Autodesk Inventor part; units mm, degrees
(part 5 of 16)
  spline S25 degree 3 poles (-39.1458, 73.8476) (-39.0245, 73.9067) (-38.9024, 73.9639) (-38.7794, 74.0192) (-38.7128, 74.0491) (-38.6461, 74.0784) (-38.5791, 74.1071) (-38.5156, 74.1342) (-38.4519, 74.1608) (-38.388, 74.1869) (-38.3277, 74.2114) (-38.2671, 74.2355) (-38.2064, 74.259) (-38.1493, 74.2811) (-38.0919, 74.3027) (-38.0344, 74.3237) (-37.9806, 74.3435) (-37.9265, 74.3627) (-37.8723, 74.3815) (-37.8218, 74.399) (-37.7711, 74.4161) (-37.7203, 74.4327) (-37.6731, 74.4481) (-37.6259, 74.4631) (-37.5784, 74.4776) (-37.5348, 74.491) (-37.4909, 74.5041) (-37.447, 74.5167) (-37.4068, 74.5283) (-37.3665, 74.5395) (-37.3262, 74.5503) (-37.2895, 74.5602) (-37.2528, 74.5697) (-37.216, 74.5789) (-37.183, 74.5871) (-37.1499, 74.5951) (-37.1167, 74.6027) (-37.0728, 74.6128) (-37.0288, 74.6223) (-36.9848, 74.6314) (-36.9749, 74.6334) (-36.9651, 74.6354) (-36.9552, 74.6375) (-36.9456, 74.6396) (-36.936, 74.6418) (-36.9264, 74.6441) (-36.917, 74.6463) (-36.9077, 74.6485) (-36.8984, 74.6509) (-36.8892, 74.6532) (-36.8801, 74.6556) (-36.871, 74.6581) (-36.8621, 74.6606) (-36.8531, 74.6631) (-36.8443, 74.6657) (-36.8355, 74.6683) (-36.8268, 74.671) (-36.8181, 74.6738) (-36.8095, 74.6765) (-36.801, 74.6794) (-36.7925, 74.6823) (-36.7841, 74.6852) (-36.7757, 74.6882) (-36.7673, 74.6914) (-36.759, 74.6945) (-36.7507, 74.6977) (-36.7425, 74.7011) (-36.7342, 74.7044) (-36.726, 74.7079) (-36.7179, 74.7115) (-36.7096, 74.7151) (-36.7015, 74.7189) (-36.6934, 74.7228) (-36.6851, 74.7268) (-36.677, 74.7309) (-36.6689, 74.7351) (-36.6606, 74.7395) (-36.6523, 74.7441) (-36.6442, 74.7489) (-36.6357, 74.7538) (-36.6274, 74.7589) (-36.6191, 74.7642) (-36.6105, 74.7698) (-36.6019, 74.7757) (-36.5936, 74.7817) (-36.5846, 74.7882) (-36.5758, 74.795) (-36.5673, 74.802) (-36.558, 74.8097) (-36.5489, 74.8176) (-36.5402, 74.8259) (-36.5305, 74.835) (-36.5213, 74.8445) (-36.5124, 74.8544) (-36.5025, 74.8654) (-36.4931, 74.8769) (-36.4843, 74.8888) (-36.4745, 74.9022) (-36.4653, 74.9162) (-36.457, 74.9306) (-36.4476, 74.9468) (-36.4392, 74.9636) (-36.432, 74.9809) (-36.424, 75.0001) (-36.4175, 75.0199) (-36.4123, 75.0401) (-36.4067, 75.0619) (-36.4028, 75.0843) (-36.401, 75.1067) (-36.3992, 75.1282) (-36.3993, 75.1498) (-36.3998, 75.1713) (-36.4022, 75.2779) (-36.4136, 75.3839) (-36.4198, 75.4902) (-36.426, 75.5965) (-36.427, 75.7031) (-36.437, 75.8092) (-36.439, 75.8307) (-36.4414, 75.8521) (-36.4457, 75.8732) (-36.4501, 75.8953) (-36.4566, 75.9171) (-36.4647, 75.9381) (-36.4721, 75.9576) (-36.481, 75.9765) (-36.4911, 75.9946) (-36.5003, 76.0109) (-36.5105, 76.0267) (-36.5217, 76.0417) (-36.5317, 76.055) (-36.5424, 76.0678) (-36.5538, 76.08) (-36.5639, 76.0908) (-36.5745, 76.1011) (-36.5857, 76.1109) (-36.5956, 76.1197) (-36.6059, 76.1281) (-36.6166, 76.136) (-36.6262, 76.1432) (-36.6361, 76.1501) (-36.6462, 76.1566) (-36.6555, 76.1625) (-36.665, 76.1682) (-36.6747, 76.1736) (-36.6837, 76.1787) (-36.6929, 76.1835) (-36.7021, 76.1881) (-36.7109, 76.1924) (-36.7198, 76.1965) (-36.7288, 76.2004) (-36.7374, 76.2042) (-36.7461, 76.2078) (-36.7549, 76.2112) (-36.7635, 76.2145) (-36.7721, 76.2176) (-36.7807, 76.2206) (-36.7892, 76.2236) (-36.7977, 76.2263) (-36.8063, 76.229) (-36.8148, 76.2316) (-36.8234, 76.2341) (-36.832, 76.2365) (-36.8405, 76.2388) (-36.8491, 76.2411) (-36.8578, 76.2432) (-36.8664, 76.2454) (-36.8751, 76.2474) (-36.8838, 76.2493) (-36.8926, 76.2512) (-36.9014, 76.2531) (-36.9103, 76.2548) (-36.9192, 76.2565) (-36.9282, 76.2582) (-36.9372, 76.2597) (-36.9463, 76.2613) (-36.9555, 76.2628) (-36.9646, 76.2642) (-36.9739, 76.2656) (-36.9833, 76.2669) (-36.9926, 76.2682) (-37.0022, 76.2695) (-37.0117, 76.2706) (-37.0213, 76.2717) (-37.0311, 76.2729) (-37.0409, 76.2739) (-37.0507, 76.2749) (-37.0607, 76.2758) (-37.0707, 76.2767) (-37.0807, 76.2776) (-37.1256, 76.2815) (-37.1704, 76.2857) (-37.2151, 76.2907) (-37.2489, 76.2944) (-37.2827, 76.2985) (-37.3165, 76.3028) (-37.3541, 76.3077) (-37.3917, 76.3129) (-37.4292, 76.3184) (-37.4706, 76.3244) (-37.5119, 76.3309) (-37.5532, 76.3377) (-37.5983, 76.3452) (-37.6433, 76.353) (-37.6882, 76.3613) (-37.737, 76.3702) (-37.7857, 76.3796) (-37.8343, 76.3894) (-37.8868, 76.4) (-37.9391, 76.4111) (-37.9913, 76.4226) (-38.0473, 76.4349) (-38.1032, 76.4478) (-38.159, 76.4611) (-38.2186, 76.4754) (-38.278, 76.4902) (-38.3373, 76.5055) (-38.4004, 76.5217) (-38.4633, 76.5386) (-38.5261, 76.556) (-38.5926, 76.5744) (-38.659, 76.5935) (-38.7251, 76.6131) (-38.795, 76.6338) (-38.8648, 76.6551) (-38.9343, 76.6771) (-39.0629, 76.7177) (-39.1909, 76.7604) (-39.3182, 76.8049) knots 0 0 0 0 0.057795 0.057795 0.057795 0.089038 0.089038 0.089038 0.118617 0.118617 0.118617 0.14653 0.14653 0.14653 0.172778 0.172778 0.172778 0.19736 0.19736 0.19736 0.220277 0.220277 0.220277 0.241529 0.241529 0.241529 0.261115 0.261115 0.261115 0.279036 0.279036 0.279036 0.295292 0.295292 0.295292 0.309882 0.309882 0.309882 0.329164 0.329164 0.329164 0.333477 0.333477 0.333477 0.337694 0.337694 0.337694 0.34182 0.34182 0.34182 0.345864 0.345864 0.345864 0.349834 0.349834 0.349834 0.353742 0.353742 0.353742 0.3576 0.3576 0.3576 0.361424 0.361424 0.361424 0.365232 0.365232 0.365232 0.369048 0.369048 0.369048 0.372899 0.372899 0.372899 0.376819 0.376819 0.376819 0.380853 0.380853 0.380853 0.385052 0.385052 0.385052 0.389482 0.389482 0.389482 0.394225 0.394225 0.394225 0.399381 0.399381 0.399381 0.405067 0.405067 0.405067 0.411413 0.411413 0.411413 0.418548 0.418548 0.418548 0.426565 0.426565 0.426565 0.435472 0.435472 0.435472 0.445133 0.445133 0.445133 0.45436 0.45436 0.45436 0.5 0.5 0.5 0.54564 0.54564 0.54564 0.554867 0.554867 0.554867 0.564528 0.564528 0.564528 0.573435 0.573435 0.573435 0.581452 0.581452 0.581452 0.588587 0.588587 0.588587 0.594933 0.594933 0.594933 0.600619 0.600619 0.600619 0.605775 0.605775 0.605775 0.610518 0.610518 0.610518 0.614948 0.614948 0.614948 0.619147 0.619147 0.619147 0.623181 0.623181 0.623181 0.627101 0.627101 0.627101 0.630952 0.630952 0.630952 0.634768 0.634768 0.634768 0.638576 0.638576 0.638576 0.6424 0.6424 0.6424 0.646258 0.646258 0.646258 0.650166 0.650166 0.650166 0.654136 0.654136 0.654136 0.65818 0.65818 0.65818 0.662306 0.662306 0.662306 0.666523 0.666523 0.666523 0.670836 0.670836 0.670836 0.690118 0.690118 0.690118 0.704708 0.704708 0.704708 0.720964 0.720964 0.720964 0.738885 0.738885 0.738885 0.758471 0.758471 0.758471 0.779723 0.779723 0.779723 0.80264 0.80264 0.80264 0.827222 0.827222 0.827222 0.85347 0.85347 0.85347 0.881383 0.881383 0.881383 0.910962 0.910962 0.910962 0.942205 0.942205 0.942205 1 1 1 1
  arc A227 (-39.1458, 73.8476) -> (-39.0178, 72.6949) centre (0.0435, 77.6158) ccw
  spline S26 degree 3 poles (-38.5372, 69.7719) (-38.4228, 69.8433) (-38.3073, 69.913) (-38.1907, 69.9808) (-38.1277, 70.0175) (-38.0644, 70.0536) (-38.0007, 70.0891) (-37.9405, 70.1228) (-37.8799, 70.1559) (-37.819, 70.1885) (-37.7616, 70.2192) (-37.7039, 70.2495) (-37.646, 70.2792) (-37.5915, 70.3071) (-37.5367, 70.3346) (-37.4817, 70.3615) (-37.4302, 70.3868) (-37.3785, 70.4116) (-37.3265, 70.4359) (-37.2781, 70.4586) (-37.2295, 70.4809) (-37.1807, 70.5027) (-37.1354, 70.523) (-37.0899, 70.5428) (-37.0443, 70.5622) (-37.0023, 70.5802) (-36.9601, 70.5977) (-36.9177, 70.6149) (-36.8789, 70.6306) (-36.84, 70.6459) (-36.801, 70.6609) (-36.7656, 70.6745) (-36.7301, 70.6878) (-36.6944, 70.7008) (-36.6624, 70.7125) (-36.6304, 70.7239) (-36.5982, 70.7349) (-36.5556, 70.7496) (-36.5128, 70.7636) (-36.47, 70.7772) (-36.4604, 70.7803) (-36.4508, 70.7833) (-36.4412, 70.7864) (-36.4319, 70.7895) (-36.4226, 70.7927) (-36.4133, 70.7959) (-36.4042, 70.7991) (-36.3951, 70.8023) (-36.3861, 70.8057) (-36.3772, 70.8089) (-36.3684, 70.8123) (-36.3596, 70.8157) (-36.351, 70.8191) (-36.3424, 70.8225) (-36.3338, 70.8261) (-36.3254, 70.8296) (-36.317, 70.8332) (-36.3087, 70.8368) (-36.3004, 70.8404) (-36.2922, 70.8442) (-36.2841, 70.848) (-36.276, 70.8518) (-36.2679, 70.8556) (-36.26, 70.8596) (-36.252, 70.8636) (-36.2441, 70.8677) (-36.2363, 70.8719) (-36.2284, 70.876) (-36.2206, 70.8804) (-36.2129, 70.8848) (-36.2051, 70.8893) (-36.1974, 70.8939) (-36.1897, 70.8986) (-36.182, 70.9034) (-36.1743, 70.9083) (-36.1667, 70.9134) (-36.1588, 70.9187) (-36.1511, 70.9241) (-36.1435, 70.9296) (-36.1356, 70.9354) (-36.1279, 70.9414) (-36.1202, 70.9476) (-36.1122, 70.9541) (-36.1043, 70.9607) (-36.0966, 70.9677) (-36.0884, 70.9751) (-36.0804, 70.9827) (-36.0726, 70.9906) (-36.0641, 70.9991) (-36.056, 71.008) (-36.0482, 71.0171) (-36.0395, 71.0272) (-36.0313, 71.0377) (-36.0235, 71.0484) (-36.0148, 71.0604) (-36.0067, 71.0728) (-35.9992, 71.0856) (-35.9908, 71.0999) (-35.9831, 71.1148) (-35.9763, 71.13) (-35.9687, 71.1471) (-35.9622, 71.1647) (-35.9568, 71.1826) (-35.9509, 71.2025) (-35.9464, 71.2229) (-35.9434, 71.2435) (-35.9401, 71.2658) (-35.9385, 71.2885) (-35.9391, 71.311) (-35.9396, 71.3325) (-35.9419, 71.354) (-35.9447, 71.3753) (-35.9582, 71.4811) (-35.9806, 71.5853) (-35.9979, 71.6904) (-36.0151, 71.7954) (-36.0273, 71.9014) (-36.0483, 72.0059) (-36.0526, 72.027) (-36.0572, 72.0481) (-36.0636, 72.0686) (-36.0703, 72.0901) (-36.079, 72.1111) (-36.0893, 72.1312) (-36.0988, 72.1497) (-36.1095, 72.1676) (-36.1215, 72.1846) (-36.1324, 72.1999) (-36.1442, 72.2144) (-36.1569, 72.2282) (-36.1682, 72.2404) (-36.1802, 72.252) (-36.1928, 72.2629) (-36.204, 72.2726) (-36.2156, 72.2818) (-36.2277, 72.2904) (-36.2385, 72.2981) (-36.2496, 72.3053) (-36.261, 72.3121) (-36.2714, 72.3182) (-36.282, 72.324) (-36.2927, 72.3294) (-36.3026, 72.3344) (-36.3126, 72.3391) (-36.3228, 72.3435) (-36.3323, 72.3475) (-36.3419, 72.3514) (-36.3516, 72.3549) (-36.3608, 72.3583) (-36.3701, 72.3615) (-36.3794, 72.3644) (-36.3884, 72.3673) (-36.3974, 72.3699) (-36.4065, 72.3724) (-36.4153, 72.3748) (-36.4242, 72.377) (-36.4331, 72.3791) (-36.4419, 72.3811) (-36.4507, 72.383) (-36.4595, 72.3847) (-36.4682, 72.3865) (-36.477, 72.388) (-36.4858, 72.3895) (-36.4945, 72.391) (-36.5033, 72.3923) (-36.5121, 72.3935) (-36.521, 72.3947) (-36.5298, 72.3958) (-36.5387, 72.3968) (-36.5476, 72.3978) (-36.5566, 72.3987) (-36.5656, 72.3995) (-36.5747, 72.4003) (-36.5838, 72.401) (-36.5928, 72.4016) (-36.6021, 72.4022) (-36.6113, 72.4028) (-36.6206, 72.4032) (-36.63, 72.4036) (-36.6395, 72.404) (-36.6489, 72.4042) (-36.6585, 72.4045) (-36.6681, 72.4047) (-36.6778, 72.4048) (-36.6876, 72.4049) (-36.6974, 72.4049) (-36.7073, 72.4048) (-36.7174, 72.4047) (-36.7274, 72.4045) (-36.7375, 72.4043) (-36.7825, 72.4036) (-36.8275, 72.4031) (-36.8725, 72.4033) (-36.9065, 72.4035) (-36.9405, 72.404) (-36.9746, 72.4048) (-37.0125, 72.4057) (-37.0504, 72.407) (-37.0883, 72.4085) (-37.1301, 72.4102) (-37.1719, 72.4123) (-37.2136, 72.4148) (-37.2592, 72.4175) (-37.3048, 72.4206) (-37.3504, 72.4241) (-37.3999, 72.4279) (-37.4493, 72.4322) (-37.4986, 72.4368) (-37.5519, 72.4419) (-37.6051, 72.4474) (-37.6582, 72.4534) (-37.7152, 72.4598) (-37.7722, 72.4668) (-37.829, 72.4742) (-37.8898, 72.4822) (-37.9504, 72.4907) (-38.011, 72.4997) (-38.0755, 72.5093) (-38.1398, 72.5194) (-38.204, 72.5302) (-38.2721, 72.5416) (-38.3401, 72.5535) (-38.408, 72.5661) (-38.4796, 72.5794) (-38.5512, 72.5934) (-38.6226, 72.6079) (-38.7548, 72.6349) (-38.8865, 72.6639) (-39.0178, 72.6949) knots 0 0 0 0 0.057795 0.057795 0.057795 0.089038 0.089038 0.089038 0.118617 0.118617 0.118617 0.14653 0.14653 0.14653 0.172778 0.172778 0.172778 0.19736 0.19736 0.19736 0.220277 0.220277 0.220277 0.241529 0.241529 0.241529 0.261115 0.261115 0.261115 0.279036 0.279036 0.279036 0.295292 0.295292 0.295292 0.309882 0.309882 0.309882 0.329164 0.329164 0.329164 0.333477 0.333477 0.333477 0.337694 0.337694 0.337694 0.34182 0.34182 0.34182 0.345864 0.345864 0.345864 0.349834 0.349834 0.349834 0.353742 0.353742 0.353742 0.3576 0.3576 0.3576 0.361424 0.361424 0.361424 0.365232 0.365232 0.365232 0.369048 0.369048 0.369048 0.372899 0.372899 0.372899 0.376819 0.376819 0.376819 0.380853 0.380853 0.380853 0.385052 0.385052 0.385052 0.389482 0.389482 0.389482 0.394225 0.394225 0.394225 0.399381 0.399381 0.399381 0.405067 0.405067 0.405067 0.411413 0.411413 0.411413 0.418548 0.418548 0.418548 0.426565 0.426565 0.426565 0.435472 0.435472 0.435472 0.445133 0.445133 0.445133 0.45436 0.45436 0.45436 0.5 0.5 0.5 0.54564 0.54564 0.54564 0.554867 0.554867 0.554867 0.564528 0.564528 0.564528 0.573435 0.573435 0.573435 0.581452 0.581452 0.581452 0.588587 0.588587 0.588587 0.594933 0.594933 0.594933 0.600619 0.600619 0.600619 0.605775 0.605775 0.605775 0.610518 0.610518 0.610518 0.614948 0.614948 0.614948 0.619147 0.619147 0.619147 0.623181 0.623181 0.623181 0.627101 0.627101 0.627101 0.630952 0.630952 0.630952 0.634768 0.634768 0.634768 0.638576 0.638576 0.638576 0.6424 0.6424 0.6424 0.646258 0.646258 0.646258 0.650166 0.650166 0.650166 0.654136 0.654136 0.654136 0.65818 0.65818 0.65818 0.662306 0.662306 0.662306 0.666523 0.666523 0.666523 0.670836 0.670836 0.670836 0.690118 0.690118 0.690118 0.704708 0.704708 0.704708 0.720964 0.720964 0.720964 0.738885 0.738885 0.738885 0.758471 0.758471 0.758471 0.779723 0.779723 0.779723 0.80264 0.80264 0.80264 0.827222 0.827222 0.827222 0.85347 0.85347 0.85347 0.881383 0.881383 0.881383 0.910962 0.910962 0.910962 0.942205 0.942205 0.942205 1 1 1 1
  arc A228 (-38.5372, 69.7719) -> (-38.2894, 68.6389) centre (0.0435, 77.6158) ccw
  spline S27 degree 3 poles (-37.5059, 65.7821) (-37.3996, 65.865) (-37.292, 65.9464) (-37.1832, 66.026) (-37.1244, 66.0691) (-37.0652, 66.1116) (-37.0056, 66.1537) (-36.9491, 66.1934) (-36.8924, 66.2327) (-36.8353, 66.2714) (-36.7814, 66.308) (-36.7272, 66.3441) (-36.6726, 66.3797) (-36.6213, 66.4132) (-36.5697, 66.4463) (-36.5179, 66.4788) (-36.4693, 66.5093) (-36.4204, 66.5394) (-36.3713, 66.569) (-36.3255, 66.5967) (-36.2795, 66.6239) (-36.2332, 66.6507) (-36.1903, 66.6756) (-36.1472, 66.7001) (-36.1039, 66.7242) (-36.0639, 66.7464) (-36.0238, 66.7682) (-35.9834, 66.7897) (-35.9465, 66.8094) (-35.9094, 66.8287) (-35.8722, 66.8477) (-35.8384, 66.865) (-35.8045, 66.8819) (-35.7704, 66.8986) (-35.7398, 66.9135) (-35.7091, 66.9282) (-35.6782, 66.9425) (-35.6374, 66.9615) (-35.5963, 66.9799) (-35.5551, 66.998) (-35.5459, 67.002) (-35.5367, 67.006) (-35.5275, 67.0102) (-35.5185, 67.0142) (-35.5096, 67.0183) (-35.5007, 67.0225) (-35.492, 67.0266) (-35.4833, 67.0308) (-35.4747, 67.0351) (-35.4662, 67.0392) (-35.4578, 67.0435) (-35.4494, 67.0478) (-35.4412, 67.0521) (-35.433, 67.0564) (-35.4248, 67.0608) (-35.4168, 67.0652) (-35.4088, 67.0696) (-35.4009, 67.0741) (-35.3931, 67.0786) (-35.3853, 67.0831) (-35.3776, 67.0878) (-35.37, 67.0924) (-35.3624, 67.0971) (-35.3549, 67.1019) (-35.3474, 67.1067) (-35.34, 67.1115) (-35.3326, 67.1165) (-35.3252, 67.1215) (-35.3179, 67.1266) (-35.3107, 67.1318) (-35.3034, 67.1371) (-35.2962, 67.1425) (-35.2891, 67.148) (-35.2819, 67.1536) (-35.2747, 67.1593) (-35.2677, 67.1652) (-35.2605, 67.1712) (-35.2534, 67.1774) (-35.2464, 67.1837) (-35.2392, 67.1903) (-35.232, 67.197) (-35.2251, 67.204) (-35.2178, 67.2112) (-35.2106, 67.2187) (-35.2037, 67.2264) (-35.1963, 67.2346) (-35.1891, 67.2431) (-35.1822, 67.2517) (-35.1747, 67.2611) (-35.1675, 67.2708) (-35.1607, 67.2807) (-35.1532, 67.2916) (-35.1461, 67.3028) (-35.1395, 67.3144) (-35.1321, 67.3272) (-35.1253, 67.3404) (-35.1192, 67.3539) (-35.1123, 67.369) (-35.1062, 67.3846) (-35.1011, 67.4004) (-35.0953, 67.4182) (-35.0906, 67.4364) (-35.0871, 67.4548) (-35.0833, 67.4752) (-35.081, 67.496) (-35.0801, 67.5168) (-35.0792, 67.5393) (-35.08, 67.562) (-35.0829, 67.5843) (-35.0857, 67.6057) (-35.0903, 67.6268) (-35.0952, 67.6477) (-35.1197, 67.7515) (-35.1529, 67.8528) (-35.1811, 67.9555) (-35.2092, 68.0582) (-35.2324, 68.1622) (-35.2642, 68.264) (-35.2707, 68.2846) (-35.2775, 68.305) (-35.286, 68.3248) (-35.2949, 68.3455) (-35.3058, 68.3654) (-35.3181, 68.3843) (-35.3294, 68.4018) (-35.342, 68.4184) (-35.3557, 68.4341) (-35.3681, 68.4481) (-35.3813, 68.4614) (-35.3954, 68.4737) (-35.4079, 68.4847) (-35.4211, 68.495) (-35.4347, 68.5045) (-35.4469, 68.513) (-35.4594, 68.5209) (-35.4723, 68.5282) (-35.4839, 68.5347) (-35.4957, 68.5407) (-35.5078, 68.5463) (-35.5187, 68.5513) (-35.5298, 68.556) (-35.5411, 68.5602) (-35.5514, 68.5641) (-35.5619, 68.5677) (-35.5725, 68.571) (-35.5823, 68.5741) (-35.5923, 68.5769) (-35.6023, 68.5794) (-35.6118, 68.5818) (-35.6214, 68.584) (-35.631, 68.586) (-35.6402, 68.5879) (-35.6495, 68.5895) (-35.6588, 68.591) (-35.6678, 68.5925) (-35.6769, 68.5938) (-35.6859, 68.5949) (-35.6949, 68.596) (-35.7038, 68.597) (-35.7127, 68.5978) (-35.7216, 68.5986) (-35.7305, 68.5993) (-35.7394, 68.5998) (-35.7482, 68.6003) (-35.7571, 68.6007) (-35.766, 68.601) (-35.7749, 68.6013) (-35.7838, 68.6015) (-35.7928, 68.6015) (-35.8018, 68.6016) (-35.8108, 68.6015) (-35.8198, 68.6014) (-35.8289, 68.6012) (-35.838, 68.601) (-35.8471, 68.6006) (-35.8564, 68.6003) (-35.8656, 68.5998) (-35.8749, 68.5993) (-35.8843, 68.5988) (-35.8937, 68.5981) (-35.9031, 68.5974) (-35.9127, 68.5966) (-35.9223, 68.5958) (-35.9319, 68.5949) (-35.9417, 68.594) (-35.9515, 68.593) (-35.9613, 68.5918) (-35.9713, 68.5907) (-35.9813, 68.5895) (-35.9912, 68.5882) (-36.0359, 68.5828) (-36.0806, 68.5776) (-36.1254, 68.5731) (-36.1593, 68.5697) (-36.1932, 68.5667) (-36.2271, 68.5639) (-36.2649, 68.5609) (-36.3027, 68.5581) (-36.3406, 68.5557) (-36.3823, 68.5531) (-36.4241, 68.5508) (-36.4659, 68.5489) (-36.5115, 68.5468) (-36.5572, 68.5451) (-36.6029, 68.5438) (-36.6525, 68.5424) (-36.7021, 68.5415) (-36.7516, 68.541) (-36.8051, 68.5404) (-36.8586, 68.5404) (-36.9121, 68.5408) (-36.9694, 68.5412) (-37.0268, 68.5422) (-37.0841, 68.5436) (-37.1454, 68.5452) (-37.2066, 68.5473) (-37.2678, 68.5499) (-37.3329, 68.5527) (-37.3979, 68.5561) (-37.4629, 68.5601) (-37.5318, 68.5643) (-37.6007, 68.5691) (-37.6695, 68.5745) (-37.7422, 68.5802) (-37.8148, 68.5866) (-37.8874, 68.5937) (-38.0216, 68.6066) (-38.1556, 68.6218) (-38.2894, 68.6389) knots 0 0 0 0 0.057795 0.057795 0.057795 0.089038 0.089038 0.089038 0.118617 0.118617 0.118617 0.14653 0.14653 0.14653 0.172778 0.172778 0.172778 0.19736 0.19736 0.19736 0.220277 0.220277 0.220277 0.241529 0.241529 0.241529 0.261115 0.261115 0.261115 0.279036 0.279036 0.279036 0.295292 0.295292 0.295292 0.309882 0.309882 0.309882 0.329164 0.329164 0.329164 0.333477 0.333477 0.333477 0.337694 0.337694 0.337694 0.34182 0.34182 0.34182 0.345864 0.345864 0.345864 0.349834 0.349834 0.349834 0.353742 0.353742 0.353742 0.3576 0.3576 0.3576 0.361424 0.361424 0.361424 0.365232 0.365232 0.365232 0.369048 0.369048 0.369048 0.372899 0.372899 0.372899 0.376819 0.376819 0.376819 0.380853 0.380853 0.380853 0.385052 0.385052 0.385052 0.389482 0.389482 0.389482 0.394225 0.394225 0.394225 0.399381 0.399381 0.399381 0.405067 0.405067 0.405067 0.411413 0.411413 0.411413 0.418548 0.418548 0.418548 0.426565 0.426565 0.426565 0.435472 0.435472 0.435472 0.445133 0.445133 0.445133 0.45436 0.45436 0.45436 0.5 0.5 0.5 0.54564 0.54564 0.54564 0.554867 0.554867 0.554867 0.564528 0.564528 0.564528 0.573435 0.573435 0.573435 0.581452 0.581452 0.581452 0.588587 0.588587 0.588587 0.594933 0.594933 0.594933 0.600619 0.600619 0.600619 0.605775 0.605775 0.605775 0.610518 0.610518 0.610518 0.614948 0.614948 0.614948 0.619147 0.619147 0.619147 0.623181 0.623181 0.623181 0.627101 0.627101 0.627101 0.630952 0.630952 0.630952 0.634768 0.634768 0.634768 0.638576 0.638576 0.638576 0.6424 0.6424 0.6424 0.646258 0.646258 0.646258 0.650166 0.650166 0.650166 0.654136 0.654136 0.654136 0.65818 0.65818 0.65818 0.662306 0.662306 0.662306 0.666523 0.666523 0.666523 0.670836 0.670836 0.670836 0.690118 0.690118 0.690118 0.704708 0.704708 0.704708 0.720964 0.720964 0.720964 0.738885 0.738885 0.738885 0.758471 0.758471 0.758471 0.779723 0.779723 0.779723 0.80264 0.80264 0.80264 0.827222 0.827222 0.827222 0.85347 0.85347 0.85347 0.881383 0.881383 0.881383 0.910962 0.910962 0.910962 0.942205 0.942205 0.942205 1 1 1 1
  arc A229 (-37.5059, 65.7821) -> (-37.1411, 64.6811) centre (0.0435, 77.6158) ccw
  spline S28 degree 3 poles (-36.0633, 61.9219) (-35.9662, 62.0155) (-35.8677, 62.1077) (-35.7678, 62.1983) (-35.7138, 62.2473) (-35.6594, 62.2958) (-35.6045, 62.3438) (-35.5525, 62.3892) (-35.5002, 62.4342) (-35.4474, 62.4787) (-35.3977, 62.5207) (-35.3475, 62.5623) (-35.297, 62.6034) (-35.2495, 62.6421) (-35.2016, 62.6803) (-35.1535, 62.7181) (-35.1083, 62.7535) (-35.0629, 62.7886) (-35.0171, 62.8232) (-34.9745, 62.8554) (-34.9316, 62.8873) (-34.8883, 62.9188) (-34.8483, 62.948) (-34.8079, 62.9769) (-34.7674, 63.0054) (-34.7299, 63.0317) (-34.6923, 63.0576) (-34.6544, 63.0832) (-34.6198, 63.1066) (-34.5849, 63.1297) (-34.5499, 63.1525) (-34.5181, 63.1732) (-34.4861, 63.1936) (-34.4539, 63.2137) (-34.4251, 63.2318) (-34.3961, 63.2496) (-34.3669, 63.2671) (-34.3283, 63.2902) (-34.2893, 63.3128) (-34.2502, 63.3351) (-34.2415, 63.3401) (-34.2327, 63.345) (-34.224, 63.3501) (-34.2155, 63.355) (-34.2071, 63.3601) (-34.1987, 63.3652) (-34.1904, 63.3702) (-34.1822, 63.3752) (-34.1741, 63.3804) (-34.1661, 63.3854) (-34.1582, 63.3905) (-34.1503, 63.3957) (-34.1426, 63.4008) (-34.1349, 63.4059) (-34.1272, 63.4112) (-34.1197, 63.4164) (-34.1123, 63.4216) (-34.1049, 63.4269) (-34.0975, 63.4322) (-34.0903, 63.4375) (-34.0831, 63.4429) (-34.076, 63.4483) (-34.0689, 63.4538) (-34.062, 63.4593) (-34.055, 63.4649) (-34.0481, 63.4705) (-34.0413, 63.4762) (-34.0345, 63.482) (-34.0278, 63.4878) (-34.0212, 63.4937) (-34.0145, 63.4997) (-34.0079, 63.5058) (-34.0014, 63.5121) (-33.9948, 63.5184) (-33.9883, 63.5248) (-33.9819, 63.5314) (-33.9753, 63.5381) (-33.9689, 63.545) (-33.9626, 63.552) (-33.9561, 63.5594) (-33.9498, 63.5668) (-33.9436, 63.5744) (-33.937, 63.5824) (-33.9307, 63.5906) (-33.9246, 63.599) (-33.9181, 63.6079) (-33.9119, 63.6171) (-33.9059, 63.6264) (-33.8994, 63.6365) (-33.8933, 63.6469) (-33.8875, 63.6575) (-33.8812, 63.6691) (-33.8753, 63.681) (-33.8699, 63.6932) (-33.8639, 63.7067) (-33.8586, 63.7205) (-33.8539, 63.7346) (-33.8486, 63.7504) (-33.8442, 63.7665) (-33.8407, 63.7828) (-33.8368, 63.8011) (-33.8341, 63.8196) (-33.8326, 63.8383) (-33.8309, 63.859) (-33.8308, 63.8799) (-33.8321, 63.9007) (-33.8335, 63.9232) (-33.8367, 63.9456) (-33.8419, 63.9676) (-33.8469, 63.9885) (-33.8537, 64.009) (-33.8608, 64.0293) (-33.896, 64.13) (-33.9396, 64.2273) (-33.9783, 64.3264) (-34.0171, 64.4256) (-34.051, 64.5267) (-34.0933, 64.6246) (-34.1018, 64.6443) (-34.1107, 64.664) (-34.1213, 64.6828) (-34.1323, 64.7024) (-34.1452, 64.7211) (-34.1594, 64.7386) (-34.1725, 64.7548) (-34.1868, 64.77) (-34.202, 64.7841) (-34.2158, 64.7968) (-34.2304, 64.8086) (-34.2457, 64.8194) (-34.2593, 64.8291) (-34.2734, 64.8379) (-34.288, 64.846) (-34.301, 64.8531) (-34.3143, 64.8596) (-34.3279, 64.8655) (-34.34, 64.8708) (-34.3524, 64.8756) (-34.365, 64.8798) (-34.3764, 64.8837) (-34.3879, 64.8872) (-34.3996, 64.8902) (-34.4103, 64.893) (-34.4211, 64.8955) (-34.4319, 64.8977) (-34.4421, 64.8997) (-34.4523, 64.9014) (-34.4625, 64.9029) (-34.4722, 64.9043) (-34.4819, 64.9055) (-34.4917, 64.9064) (-34.5011, 64.9074) (-34.5104, 64.9081) (-34.5198, 64.9086) (-34.529, 64.9091) (-34.5381, 64.9094) (-34.5473, 64.9096) (-34.5563, 64.9098) (-34.5652, 64.9098) (-34.5742, 64.9096) (-34.5831, 64.9095) (-34.592, 64.9092) (-34.6009, 64.9088) (-34.6098, 64.9084) (-34.6187, 64.9079) (-34.6275, 64.9073) (-34.6364, 64.9066) (-34.6453, 64.9059) (-34.6542, 64.905) (-34.6632, 64.9041) (-34.6721, 64.9031) (-34.6811, 64.902) (-34.6901, 64.9009) (-34.6991, 64.8997) (-34.7082, 64.8984) (-34.7173, 64.8971) (-34.7265, 64.8957) (-34.7356, 64.8942) (-34.745, 64.8927) (-34.7543, 64.8911) (-34.7635, 64.8893) (-34.773, 64.8876) (-34.7825, 64.8858) (-34.7919, 64.8839) (-34.8015, 64.8819) (-34.8112, 64.8799) (-34.8208, 64.8778) (-34.8306, 64.8756) (-34.8404, 64.8733) (-34.8502, 64.871) (-34.8941, 64.8609) (-34.938, 64.8511) (-34.982, 64.842) (-35.0154, 64.8351) (-35.0488, 64.8285) (-35.0822, 64.8222) (-35.1195, 64.8152) (-35.1569, 64.8085) (-35.1943, 64.8022) (-35.2355, 64.7952) (-35.2768, 64.7885) (-35.3181, 64.7823) (-35.3633, 64.7754) (-35.4086, 64.769) (-35.4539, 64.7629) (-35.503, 64.7564) (-35.5522, 64.7503) (-35.6015, 64.7446) (-35.6546, 64.7384) (-35.7078, 64.7328) (-35.761, 64.7276) (-35.8181, 64.722) (-35.8753, 64.717) (-35.9325, 64.7124) (-35.9935, 64.7076) (-36.0546, 64.7033) (-36.1157, 64.6995) (-36.1808, 64.6955) (-36.2458, 64.6921) (-36.3109, 64.6892) (-36.3798, 64.6862) (-36.4488, 64.6838) (-36.5178, 64.682) (-36.5907, 64.6801) (-36.6636, 64.6788) (-36.7365, 64.6782) (-36.8714, 64.6771) (-37.0062, 64.6781) (-37.1411, 64.6811) knots 0 0 0 0 0.057795 0.057795 0.057795 0.089038 0.089038 0.089038 0.118617 0.118617 0.118617 0.14653 0.14653 0.14653 0.172778 0.172778 0.172778 0.19736 0.19736 0.19736 0.220277 0.220277 0.220277 0.241529 0.241529 0.241529 0.261115 0.261115 0.261115 0.279036 0.279036 0.279036 0.295292 0.295292 0.295292 0.309882 0.309882 0.309882 0.329164 0.329164 0.329164 0.333477 0.333477 0.333477 0.337694 0.337694 0.337694 0.34182 0.34182 0.34182 0.345864 0.345864 0.345864 0.349834 0.349834 0.349834 0.353742 0.353742 0.353742 0.3576 0.3576 0.3576 0.361424 0.361424 0.361424 0.365232 0.365232 0.365232 0.369048 0.369048 0.369048 0.372899 0.372899 0.372899 0.376819 0.376819 0.376819 0.380853 0.380853 0.380853 0.385052 0.385052 0.385052 0.389482 0.389482 0.389482 0.394225 0.394225 0.394225 0.399381 0.399381 0.399381 0.405067 0.405067 0.405067 0.411413 0.411413 0.411413 0.418548 0.418548 0.418548 0.426565 0.426565 0.426565 0.435472 0.435472 0.435472 0.445133 0.445133 0.445133 0.45436 0.45436 0.45436 0.5 0.5 0.5 0.54564 0.54564 0.54564 0.554867 0.554867 0.554867 0.564528 0.564528 0.564528 0.573435 0.573435 0.573435 0.581452 0.581452 0.581452 0.588587 0.588587 0.588587 0.594933 0.594933 0.594933 0.600619 0.600619 0.600619 0.605775 0.605775 0.605775 0.610518 0.610518 0.610518 0.614948 0.614948 0.614948 0.619147 0.619147 0.619147 0.623181 0.623181 0.623181 0.627101 0.627101 0.627101 0.630952 0.630952 0.630952 0.634768 0.634768 0.634768 0.638576 0.638576 0.638576 0.6424 0.6424 0.6424 0.646258 0.646258 0.646258 0.650166 0.650166 0.650166 0.654136 0.654136 0.654136 0.65818 0.65818 0.65818 0.662306 0.662306 0.662306 0.666523 0.666523 0.666523 0.670836 0.670836 0.670836 0.690118 0.690118 0.690118 0.704708 0.704708 0.704708 0.720964 0.720964 0.720964 0.738885 0.738885 0.738885 0.758471 0.758471 0.758471 0.779723 0.779723 0.779723 0.80264 0.80264 0.80264 0.827222 0.827222 0.827222 0.85347 0.85347 0.85347 0.881383 0.881383 0.881383 0.910962 0.910962 0.910962 0.942205 0.942205 0.942205 1 1 1 1
  arc A230 (-36.0633, 61.9219) -> (-35.5853, 60.8652) centre (0.0435, 77.6158) ccw
  spline S29 degree 3 poles (-34.225, 58.2337) (-34.1383, 58.3369) (-34.05, 58.4389) (-33.9601, 58.5394) (-33.9115, 58.5938) (-33.8624, 58.6477) (-33.8128, 58.7012) (-33.7659, 58.7518) (-33.7186, 58.802) (-33.6708, 58.8518) (-33.6256, 58.8988) (-33.5801, 58.9454) (-33.5342, 58.9916) (-33.491, 59.035) (-33.4474, 59.078) (-33.4034, 59.1207) (-33.3622, 59.1606) (-33.3207, 59.2002) (-33.2788, 59.2394) (-33.2398, 59.2759) (-33.2004, 59.3121) (-33.1607, 59.348) (-33.1239, 59.3812) (-33.0868, 59.4141) (-33.0495, 59.4467) (-33.015, 59.4767) (-32.9803, 59.5065) (-32.9453, 59.5359) (-32.9133, 59.5628) (-32.881, 59.5894) (-32.8485, 59.6157) (-32.8191, 59.6396) (-32.7894, 59.6633) (-32.7595, 59.6866) (-32.7327, 59.7076) (-32.7057, 59.7284) (-32.6785, 59.7488) (-32.6425, 59.7759) (-32.6062, 59.8024) (-32.5696, 59.8286) (-32.5615, 59.8345) (-32.5533, 59.8404) (-32.5452, 59.8463) (-32.5372, 59.8521) (-32.5293, 59.858) (-32.5215, 59.864) (-32.5138, 59.8698) (-32.5062, 59.8757) (-32.4987, 59.8816) (-32.4912, 59.8875) (-32.4839, 59.8934) (-32.4766, 59.8994) (-32.4694, 59.9052) (-32.4623, 59.9112) (-32.4553, 59.9172) (-32.4483, 59.9231) (-32.4415, 59.9291) (-32.4346, 59.9352) (-32.4279, 59.9412) (-32.4213, 59.9472) (-32.4147, 59.9534) (-32.4082, 59.9595) (-32.4017, 59.9657) (-32.3954, 59.9719) (-32.389, 59.9781) (-32.3828, 59.9845) (-32.3766, 59.9909) (-32.3705, 59.9973) (-32.3644, 60.0038) (-32.3584, 60.0104) (-32.3524, 60.017) (-32.3464, 60.0238) (-32.3406, 60.0307) (-32.3347, 60.0376) (-32.3289, 60.0447) (-32.3233, 60.0519) (-32.3175, 60.0593) (-32.3118, 60.0668) (-32.3063, 60.0745) (-32.3006, 60.0824) (-32.295, 60.0905) (-32.2897, 60.0987) (-32.284, 60.1074) (-32.2786, 60.1162) (-32.2734, 60.1251) (-32.2679, 60.1347) (-32.2626, 60.1445) (-32.2576, 60.1544) (-32.2523, 60.1651) (-32.2472, 60.1761) (-32.2426, 60.1872) (-32.2375, 60.1994) (-32.2329, 60.2119) (-32.2288, 60.2245) (-32.2243, 60.2386) (-32.2204, 60.2529) (-32.2172, 60.2674) (-32.2136, 60.2837) (-32.2109, 60.3001) (-32.2092, 60.3167) (-32.2072, 60.3353) (-32.2064, 60.3541) (-32.2069, 60.3728) (-32.2074, 60.3936) (-32.2094, 60.4143) (-32.2129, 60.4348) (-32.2167, 60.4571) (-32.2222, 60.4791) (-32.2297, 60.5004) (-32.2368, 60.5207) (-32.2457, 60.5403) (-32.2549, 60.5598) (-32.3004, 60.6562) (-32.3539, 60.7484) (-32.4028, 60.843) (-32.4517, 60.9376) (-32.496, 61.0346) (-32.5483, 61.1275) (-32.5589, 61.1462) (-32.5698, 61.1649) (-32.5823, 61.1824) (-32.5953, 61.2008) (-32.61, 61.218) (-32.626, 61.234) (-32.6407, 61.2487) (-32.6565, 61.2624) (-32.6732, 61.2748) (-32.6882, 61.286) (-32.7039, 61.2962) (-32.7202, 61.3053) (-32.7348, 61.3135) (-32.7498, 61.3208) (-32.7651, 61.3273) (-32.7788, 61.3331) (-32.7927, 61.3382) (-32.8068, 61.3426) (-32.8195, 61.3466) (-32.8323, 61.35) (-32.8452, 61.3529) (-32.857, 61.3556) (-32.8688, 61.3578) (-32.8807, 61.3597) (-32.8917, 61.3613) (-32.9026, 61.3627) (-32.9137, 61.3637) (-32.924, 61.3646) (-32.9343, 61.3653) (-32.9446, 61.3657) (-32.9544, 61.3661) (-32.9642, 61.3662) (-32.974, 61.3662) (-32.9834, 61.3661) (-32.9928, 61.3658) (-33.0022, 61.3653) (-33.0114, 61.3649) (-33.0205, 61.3643) (-33.0296, 61.3635) (-33.0386, 61.3627) (-33.0475, 61.3618) (-33.0564, 61.3607) (-33.0653, 61.3597) (-33.0741, 61.3585) (-33.0829, 61.3571) (-33.0917, 61.3558) (-33.1005, 61.3544) (-33.1092, 61.3528) (-33.118, 61.3512) (-33.1268, 61.3495) (-33.1355, 61.3477) (-33.1443, 61.3459) (-33.1531, 61.344) (-33.1619, 61.342) (-33.1708, 61.3399) (-33.1796, 61.3378) (-33.1885, 61.3356) (-33.1975, 61.3333) (-33.2064, 61.3309) (-33.2154, 61.3285) (-33.2245, 61.326) (-33.2335, 61.3234) (-33.2426, 61.3207) (-33.2518, 61.318) (-33.261, 61.3152) (-33.2702, 61.3123) (-33.2796, 61.3094) (-33.289, 61.3064) (-33.2983, 61.3032) (-33.3078, 61.3) (-33.3174, 61.2967) (-33.3269, 61.2935) (-33.3694, 61.2788) (-33.4121, 61.2645) (-33.4549, 61.2508) (-33.4874, 61.2404) (-33.5199, 61.2304) (-33.5525, 61.2207) (-33.5889, 61.2098) (-33.6253, 61.1992) (-33.6618, 61.189) (-33.7021, 61.1777) (-33.7425, 61.1668) (-33.7829, 61.1563) (-33.8272, 61.1447) (-33.8715, 61.1336) (-33.9159, 61.1229) (-33.9641, 61.1112) (-34.0124, 61.1) (-34.0608, 61.0892) (-34.113, 61.0775) (-34.1653, 61.0663) (-34.2177, 61.0556) (-34.2739, 61.0441) (-34.3302, 61.0331) (-34.3866, 61.0226) (-34.4468, 61.0114) (-34.5071, 61.0007) (-34.5675, 60.9906) (-34.6318, 60.9798) (-34.6961, 60.9696) (-34.7605, 60.9599) (-34.8288, 60.9497) (-34.8971, 60.9401) (-34.9656, 60.9311) (-35.0379, 60.9216) (-35.1102, 60.9128) (-35.1827, 60.9045) (-35.3167, 60.8893) (-35.4509, 60.8763) (-35.5853, 60.8652) knots 0 0 0 0 0.057795 0.057795 0.057795 0.089038 0.089038 0.089038 0.118617 0.118617 0.118617 0.14653 0.14653 0.14653 0.172778 0.172778 0.172778 0.19736 0.19736 0.19736 0.220277 0.220277 0.220277 0.241529 0.241529 0.241529 0.261115 0.261115 0.261115 0.279036 0.279036 0.279036 0.295292 0.295292 0.295292 0.309882 0.309882 0.309882 0.329164 0.329164 0.329164 0.333477 0.333477 0.333477 0.337694 0.337694 0.337694 0.34182 0.34182 0.34182 0.345864 0.345864 0.345864 0.349834 0.349834 0.349834 0.353742 0.353742 0.353742 0.3576 0.3576 0.3576 0.361424 0.361424 0.361424 0.365232 0.365232 0.365232 0.369048 0.369048 0.369048 0.372899 0.372899 0.372899 0.376819 0.376819 0.376819 0.380853 0.380853 0.380853 0.385052 0.385052 0.385052 0.389482 0.389482 0.389482 0.394225 0.394225 0.394225 0.399381 0.399381 0.399381 0.405067 0.405067 0.405067 0.411413 0.411413 0.411413 0.418548 0.418548 0.418548 0.426565 0.426565 0.426565 0.435472 0.435472 0.435472 0.445133 0.445133 0.445133 0.45436 0.45436 0.45436 0.5 0.5 0.5 0.54564 0.54564 0.54564 0.554867 0.554867 0.554867 0.564528 0.564528 0.564528 0.573435 0.573435 0.573435 0.581452 0.581452 0.581452 0.588587 0.588587 0.588587 0.594933 0.594933 0.594933 0.600619 0.600619 0.600619 0.605775 0.605775 0.605775 0.610518 0.610518 0.610518 0.614948 0.614948 0.614948 0.619147 0.619147 0.619147 0.623181 0.623181 0.623181 0.627101 0.627101 0.627101 0.630952 0.630952 0.630952 0.634768 0.634768 0.634768 0.638576 0.638576 0.638576 0.6424 0.6424 0.6424 0.646258 0.646258 0.646258 0.650166 0.650166 0.650166 0.654136 0.654136 0.654136 0.65818 0.65818 0.65818 0.662306 0.662306 0.662306 0.666523 0.666523 0.666523 0.670836 0.670836 0.670836 0.690118 0.690118 0.690118 0.704708 0.704708 0.704708 0.720964 0.720964 0.720964 0.738885 0.738885 0.738885 0.758471 0.758471 0.758471 0.779723 0.779723 0.779723 0.80264 0.80264 0.80264 0.827222 0.827222 0.827222 0.85347 0.85347 0.85347 0.881383 0.881383 0.881383 0.910962 0.910962 0.910962 0.942205 0.942205 0.942205 1 1 1 1
  arc A231 (-34.225, 58.2337) -> (-33.6392, 57.2327) centre (0.0435, 77.6158) ccw
  spline S30 degree 3 poles (-32.0113, 54.7578) (-31.9358, 54.8696) (-31.8587, 54.9802) (-31.7798, 55.0896) (-31.7371, 55.1487) (-31.694, 55.2075) (-31.6503, 55.2659) (-31.6089, 55.3211) (-31.567, 55.376) (-31.5247, 55.4305) (-31.4847, 55.482) (-31.4443, 55.533) (-31.4035, 55.5838) (-31.365, 55.6315) (-31.3262, 55.6788) (-31.2869, 55.7258) (-31.2501, 55.7698) (-31.213, 55.8136) (-31.1754, 55.8569) (-31.1404, 55.8973) (-31.1051, 55.9375) (-31.0693, 55.9773) (-31.0362, 56.0142) (-31.0028, 56.0508) (-30.969, 56.0871) (-30.9379, 56.1205) (-30.9064, 56.1537) (-30.8747, 56.1866) (-30.8457, 56.2168) (-30.8164, 56.2466) (-30.7868, 56.2762) (-30.76, 56.303) (-30.733, 56.3296) (-30.7057, 56.356) (-30.6812, 56.3797) (-30.6566, 56.4031) (-30.6316, 56.4263) (-30.5987, 56.457) (-30.5653, 56.4872) (-30.5317, 56.5171) (-30.5242, 56.5238) (-30.5167, 56.5304) (-30.5092, 56.5372) (-30.5019, 56.5438) (-30.4947, 56.5505) (-30.4875, 56.5572) (-30.4805, 56.5638) (-30.4736, 56.5705) (-30.4667, 56.5772) (-30.4599, 56.5838) (-30.4532, 56.5904) (-30.4466, 56.5971) (-30.4401, 56.6037) (-30.4336, 56.6104) (-30.4272, 56.6171) (-30.4209, 56.6237) (-30.4147, 56.6304) (-30.4086, 56.6371) (-30.4025, 56.6438) (-30.3966, 56.6505) (-30.3907, 56.6573) (-30.3848, 56.6641) (-30.3791, 56.6709) (-30.3734, 56.6778) (-30.3677, 56.6846) (-30.3622, 56.6916) (-30.3567, 56.6986) (-30.3513, 56.7056) (-30.3459, 56.7127) (-30.3406, 56.7199) (-30.3353, 56.7272) (-30.3301, 56.7345) (-30.3251, 56.7419) (-30.3199, 56.7495) (-30.3149, 56.7571) (-30.31, 56.7649) (-30.305, 56.7729) (-30.3002, 56.7809) (-30.2955, 56.7891) (-30.2906, 56.7976) (-30.286, 56.8062) (-30.2815, 56.8149) (-30.2768, 56.8241) (-30.2723, 56.8335) (-30.2681, 56.8429) (-30.2636, 56.853) (-30.2594, 56.8633) (-30.2555, 56.8736) (-30.2512, 56.8849) (-30.2474, 56.8963) (-30.244, 56.9078) (-30.2402, 56.9206) (-30.2369, 56.9334) (-30.2342, 56.9464) (-30.2311, 56.9609) (-30.2287, 56.9755) (-30.2271, 56.9903) (-30.2252, 57.0068) (-30.2243, 57.0235) (-30.2242, 57.0401) (-30.2242, 57.0589) (-30.2254, 57.0776) (-30.2278, 57.0961) (-30.2305, 57.1168) (-30.2347, 57.1372) (-30.2403, 57.1572) (-30.2464, 57.179) (-30.2542, 57.2003) (-30.2638, 57.2206) (-30.273, 57.2401) (-30.2839, 57.2587) (-30.2951, 57.2772) (-30.3505, 57.3683) (-30.4133, 57.4544) (-30.4719, 57.5433) (-30.5304, 57.6323) (-30.5845, 57.7241) (-30.6463, 57.811) (-30.6588, 57.8286) (-30.6715, 57.846) (-30.6858, 57.8621) (-30.7007, 57.879) (-30.7171, 57.8946) (-30.7347, 57.9088) (-30.7509, 57.9219) (-30.768, 57.9339) (-30.7858, 57.9445) (-30.8019, 57.954) (-30.8187, 57.9625) (-30.8359, 57.9699) (-30.8512, 57.9765) (-30.8668, 57.9822) (-30.8828, 57.9871) (-30.8969, 57.9914) (-30.9113, 57.995) (-30.9258, 57.998) (-30.9389, 58.0006) (-30.952, 58.0027) (-30.9651, 58.0042) (-30.9771, 58.0056) (-30.9891, 58.0066) (-31.0011, 58.0072) (-31.0122, 58.0077) (-31.0233, 58.0079) (-31.0343, 58.0078) (-31.0447, 58.0076) (-31.055, 58.0072) (-31.0653, 58.0065) (-31.0751, 58.0059) (-31.0849, 58.005) (-31.0946, 58.0039) (-31.1039, 58.0028) (-31.1133, 58.0016) (-31.1226, 58.0001) (-31.1316, 57.9987) (-31.1406, 57.9972) (-31.1496, 57.9954) (-31.1584, 57.9937) (-31.1672, 57.9919) (-31.176, 57.9899) (-31.1847, 57.9879) (-31.1933, 57.9858) (-31.2019, 57.9835) (-31.2105, 57.9813) (-31.2191, 57.979) (-31.2277, 57.9765) (-31.2362, 57.974) (-31.2448, 57.9714) (-31.2533, 57.9687) (-31.2618, 57.966) (-31.2704, 57.9632) (-31.2789, 57.9602) (-31.2875, 57.9573) (-31.2961, 57.9542) (-31.3047, 57.9511) (-31.3134, 57.9479) (-31.322, 57.9446) (-31.3307, 57.9412) (-31.3395, 57.9378) (-31.3482, 57.9343) (-31.3569, 57.9307) (-31.3658, 57.927) (-31.3747, 57.9232) (-31.3835, 57.9194) (-31.3926, 57.9155) (-31.4016, 57.9115) (-31.4105, 57.9074) (-31.4197, 57.9033) (-31.4288, 57.899) (-31.4379, 57.8947) (-31.4787, 57.8757) (-31.5196, 57.857) (-31.5608, 57.8389) (-31.592, 57.8252) (-31.6233, 57.8118) (-31.6547, 57.7987) (-31.6897, 57.7841) (-31.7249, 57.7698) (-31.7601, 57.7558) (-31.799, 57.7404) (-31.838, 57.7253) (-31.8772, 57.7106) (-31.9199, 57.6945) (-31.9629, 57.6788) (-32.0059, 57.6635) (-32.0526, 57.6468) (-32.0995, 57.6306) (-32.1465, 57.6148) (-32.1972, 57.5978) (-32.248, 57.5812) (-32.299, 57.565) (-32.3537, 57.5477) (-32.4085, 57.5309) (-32.4635, 57.5146) (-32.5222, 57.4971) (-32.5811, 57.4802) (-32.6401, 57.4638) (-32.7029, 57.4464) (-32.7658, 57.4295) (-32.8289, 57.4132) (-32.8957, 57.3959) (-32.9627, 57.3792) (-33.0298, 57.3631) (-33.1007, 57.3461) (-33.1717, 57.3297) (-33.2429, 57.314) (-33.3746, 57.2848) (-33.5067, 57.2578) (-33.6392, 57.2327) knots 0 0 0 0 0.057795 0.057795 0.057795 0.089038 0.089038 0.089038 0.118617 0.118617 0.118617 0.14653 0.14653 0.14653 0.172778 0.172778 0.172778 0.19736 0.19736 0.19736 0.220277 0.220277 0.220277 0.241529 0.241529 0.241529 0.261115 0.261115 0.261115 0.279036 0.279036 0.279036 0.295292 0.295292 0.295292 0.309882 0.309882 0.309882 0.329164 0.329164 0.329164 0.333477 0.333477 0.333477 0.337694 0.337694 0.337694 0.34182 0.34182 0.34182 0.345864 0.345864 0.345864 0.349834 0.349834 0.349834 0.353742 0.353742 0.353742 0.3576 0.3576 0.3576 0.361424 0.361424 0.361424 0.365232 0.365232 0.365232 0.369048 0.369048 0.369048 0.372899 0.372899 0.372899 0.376819 0.376819 0.376819 0.380853 0.380853 0.380853 0.385052 0.385052 0.385052 0.389482 0.389482 0.389482 0.394225 0.394225 0.394225 0.399381 0.399381 0.399381 0.405067 0.405067 0.405067 0.411413 0.411413 0.411413 0.418548 0.418548 0.418548 0.426565 0.426565 0.426565 0.435472 0.435472 0.435472 0.445133 0.445133 0.445133 0.45436 0.45436 0.45436 0.5 0.5 0.5 0.54564 0.54564 0.54564 0.554867 0.554867 0.554867 0.564528 0.564528 0.564528 0.573435 0.573435 0.573435 0.581452 0.581452 0.581452 0.588587 0.588587 0.588587 0.594933 0.594933 0.594933 0.600619 0.600619 0.600619 0.605775 0.605775 0.605775 0.610518 0.610518 0.610518 0.614948 0.614948 0.614948 0.619147 0.619147 0.619147 0.623181 0.623181 0.623181 0.627101 0.627101 0.627101 0.630952 0.630952 0.630952 0.634768 0.634768 0.634768 0.638576 0.638576 0.638576 0.6424 0.6424 0.6424 0.646258 0.646258 0.646258 0.650166 0.650166 0.650166 0.654136 0.654136 0.654136 0.65818 0.65818 0.65818 0.662306 0.662306 0.662306 0.666523 0.666523 0.666523 0.670836 0.670836 0.670836 0.690118 0.690118 0.690118 0.704708 0.704708 0.704708 0.720964 0.720964 0.720964 0.738885 0.738885 0.738885 0.758471 0.758471 0.758471 0.779723 0.779723 0.779723 0.80264 0.80264 0.80264 0.827222 0.827222 0.827222 0.85347 0.85347 0.85347 0.881383 0.881383 0.881383 0.910962 0.910962 0.910962 0.942205 0.942205 0.942205 1 1 1 1
  arc A232 (-32.0113, 54.7578) -> (-31.3241, 53.8236) centre (0.0435, 77.6158) ccw
  spline S31 degree 3 poles (-29.4464, 51.5324) (-29.383, 51.6514) (-29.3179, 51.7695) (-29.2508, 51.8866) (-29.2146, 51.9498) (-29.1778, 52.0128) (-29.1404, 52.0754) (-29.1051, 52.1347) (-29.0692, 52.1936) (-29.0328, 52.2523) (-28.9984, 52.3076) (-28.9636, 52.3626) (-28.9282, 52.4174) (-28.895, 52.4688) (-28.8613, 52.52) (-28.8272, 52.5708) (-28.7952, 52.6184) (-28.7628, 52.6658) (-28.73, 52.7128) (-28.6994, 52.7567) (-28.6684, 52.8003) (-28.6371, 52.8436) (-28.608, 52.8838) (-28.5785, 52.9237) (-28.5487, 52.9633) (-28.5213, 52.9999) (-28.4935, 53.0362) (-28.4654, 53.0722) (-28.4397, 53.1052) (-28.4137, 53.1379) (-28.3874, 53.1705) (-28.3635, 53.1999) (-28.3394, 53.2292) (-28.315, 53.2583) (-28.2931, 53.2844) (-28.2711, 53.3103) (-28.2487, 53.336) (-28.2191, 53.3699) (-28.1891, 53.4034) (-28.1588, 53.4367) (-28.152, 53.4441) (-28.1452, 53.4515) (-28.1385, 53.459) (-28.132, 53.4664) (-28.1255, 53.4738) (-28.1191, 53.4812) (-28.1128, 53.4885) (-28.1066, 53.4959) (-28.1004, 53.5033) (-28.0944, 53.5105) (-28.0884, 53.5178) (-28.0825, 53.5252) (-28.0767, 53.5324) (-28.071, 53.5397) (-28.0653, 53.5471) (-28.0598, 53.5543) (-28.0543, 53.5616) (-28.0489, 53.569) (-28.0436, 53.5762) (-28.0384, 53.5835) (-28.0332, 53.5909) (-28.0281, 53.5982) (-28.0231, 53.6056) (-28.0181, 53.613) (-28.0132, 53.6205) (-28.0084, 53.6279) (-28.0037, 53.6355) (-27.999, 53.643) (-27.9944, 53.6507) (-27.99, 53.6584) (-27.9855, 53.6661) (-27.9811, 53.674) (-27.9768, 53.6819) (-27.9725, 53.69) (-27.9683, 53.6981) (-27.9643, 53.7063) (-27.9601, 53.7148) (-27.9561, 53.7233) (-27.9523, 53.7319) (-27.9484, 53.7409) (-27.9446, 53.7499) (-27.9411, 53.7591) (-27.9374, 53.7687) (-27.9339, 53.7785) (-27.9307, 53.7883) (-27.9273, 53.7988) (-27.9241, 53.8094) (-27.9214, 53.8201) (-27.9183, 53.8318) (-27.9157, 53.8435) (-27.9135, 53.8554) (-27.911, 53.8684) (-27.9091, 53.8816) (-27.9078, 53.8948) (-27.9062, 53.9095) (-27.9054, 53.9243) (-27.9053, 53.9391) (-27.9052, 53.9558) (-27.906, 53.9724) (-27.9077, 53.989) (-27.9096, 54.0076) (-27.9128, 54.0261) (-27.9171, 54.0443) (-27.9219, 54.0646) (-27.9282, 54.0844) (-27.9359, 54.1038) (-27.9442, 54.1248) (-27.9542, 54.1451) (-27.9659, 54.1644) (-27.9771, 54.1828) (-27.9899, 54.2002) (-28.0029, 54.2173) (-28.0675, 54.3022) (-28.1391, 54.3812) (-28.2066, 54.4636) (-28.274, 54.5459) (-28.3375, 54.6316) (-28.408, 54.7116) (-28.4222, 54.7277) (-28.4368, 54.7437) (-28.4526, 54.7583) (-28.4692, 54.7735) (-28.4872, 54.7873) (-28.5061, 54.7996) (-28.5236, 54.8109) (-28.5418, 54.821) (-28.5607, 54.8297) (-28.5777, 54.8375) (-28.5953, 54.8442) (-28.6131, 54.8498) (-28.6291, 54.8547) (-28.6452, 54.8588) (-28.6616, 54.8619) (-28.6761, 54.8647) (-28.6908, 54.8668) (-28.7056, 54.8682) (-28.7188, 54.8695) (-28.732, 54.8702) (-28.7453, 54.8704) (-28.7573, 54.8705) (-28.7694, 54.8703) (-28.7814, 54.8696) (-28.7925, 54.8689) (-28.8035, 54.868) (-28.8145, 54.8667) (-28.8247, 54.8654) (-28.835, 54.864) (-28.8452, 54.8622) (-28.8548, 54.8605) (-28.8644, 54.8586) (-28.874, 54.8565) (-28.8832, 54.8545) (-28.8924, 54.8523) (-28.9015, 54.8499) (-28.9103, 54.8475) (-28.9191, 54.845) (-28.9279, 54.8424) (-28.9364, 54.8397) (-28.945, 54.837) (-28.9535, 54.8341) (-28.9619, 54.8312) (-28.9703, 54.8282) (-28.9787, 54.8251) (-28.987, 54.8219) (-28.9952, 54.8187) (-29.0035, 54.8153) (-29.0117, 54.812) (-29.02, 54.8085) (-29.0281, 54.8049) (-29.0364, 54.8013) (-29.0446, 54.7976) (-29.0528, 54.7938) (-29.061, 54.79) (-29.0693, 54.786) (-29.0774, 54.782) (-29.0858, 54.7779) (-29.094, 54.7738) (-29.1023, 54.7695) (-29.1106, 54.7652) (-29.119, 54.7608) (-29.1273, 54.7563) (-29.1357, 54.7517) (-29.1442, 54.747) (-29.1526, 54.7423) (-29.1611, 54.7374) (-29.1697, 54.7325) (-29.1781, 54.7276) (-29.1868, 54.7224) (-29.1954, 54.7172) (-29.2041, 54.7121) (-29.2426, 54.6889) (-29.2814, 54.666) (-29.3204, 54.6437) (-29.35, 54.6268) (-29.3798, 54.6103) (-29.4096, 54.5939) (-29.4429, 54.5757) (-29.4764, 54.5579) (-29.51, 54.5403) (-29.547, 54.5208) (-29.5842, 54.5018) (-29.6216, 54.483) (-29.6625, 54.4626) (-29.7035, 54.4425) (-29.7448, 54.4227) (-29.7895, 54.4013) (-29.8344, 54.3802) (-29.8795, 54.3596) (-29.9281, 54.3374) (-29.9769, 54.3156) (-30.026, 54.2942) (-30.0785, 54.2712) (-30.1313, 54.2488) (-30.1843, 54.2268) (-30.2409, 54.2033) (-30.2977, 54.1803) (-30.3546, 54.1578) (-30.4152, 54.1339) (-30.476, 54.1106) (-30.537, 54.0878) (-30.6017, 54.0636) (-30.6666, 54.04) (-30.7316, 54.0169) (-30.8003, 53.9926) (-30.8693, 53.9689) (-30.9384, 53.9458) (-31.0664, 53.903) (-31.195, 53.8624) (-31.3241, 53.8236) knots 0 0 0 0 0.057795 0.057795 0.057795 0.089038 0.089038 0.089038 0.118617 0.118617 0.118617 0.14653 0.14653 0.14653 0.172778 0.172778 0.172778 0.19736 0.19736 0.19736 0.220277 0.220277 0.220277 0.241529 0.241529 0.241529 0.261115 0.261115 0.261115 0.279036 0.279036 0.279036 0.295292 0.295292 0.295292 0.309882 0.309882 0.309882 0.329164 0.329164 0.329164 0.333477 0.333477 0.333477 0.337694 0.337694 0.337694 0.34182 0.34182 0.34182 0.345864 0.345864 0.345864 0.349834 0.349834 0.349834 0.353742 0.353742 0.353742 0.3576 0.3576 0.3576 0.361424 0.361424 0.361424 0.365232 0.365232 0.365232 0.369048 0.369048 0.369048 0.372899 0.372899 0.372899 0.376819 0.376819 0.376819 0.380853 0.380853 0.380853 0.385052 0.385052 0.385052 0.389482 0.389482 0.389482 0.394225 0.394225 0.394225 0.399381 0.399381 0.399381 0.405067 0.405067 0.405067 0.411413 0.411413 0.411413 0.418548 0.418548 0.418548 0.426565 0.426565 0.426565 0.435472 0.435472 0.435472 0.445133 0.445133 0.445133 0.45436 0.45436 0.45436 0.5 0.5 0.5 0.54564 0.54564 0.54564 0.554867 0.554867 0.554867 0.564528 0.564528 0.564528 0.573435 0.573435 0.573435 0.581452 0.581452 0.581452 0.588587 0.588587 0.588587 0.594933 0.594933 0.594933 0.600619 0.600619 0.600619 0.605775 0.605775 0.605775 0.610518 0.610518 0.610518 0.614948 0.614948 0.614948 0.619147 0.619147 0.619147 0.623181 0.623181 0.623181 0.627101 0.627101 0.627101 0.630952 0.630952 0.630952 0.634768 0.634768 0.634768 0.638576 0.638576 0.638576 0.6424 0.6424 0.6424 0.646258 0.646258 0.646258 0.650166 0.650166 0.650166 0.654136 0.654136 0.654136 0.65818 0.65818 0.65818 0.662306 0.662306 0.662306 0.666523 0.666523 0.666523 0.670836 0.670836 0.670836 0.690118 0.690118 0.690118 0.704708 0.704708 0.704708 0.720964 0.720964 0.720964 0.738885 0.738885 0.738885 0.758471 0.758471 0.758471 0.779723 0.779723 0.779723 0.80264 0.80264 0.80264 0.827222 0.827222 0.827222 0.85347 0.85347 0.85347 0.881383 0.881383 0.881383 0.910962 0.910962 0.910962 0.942205 0.942205 0.942205 1 1 1 1
  arc A233 (-29.4464, 51.5324) -> (-28.6653, 50.6751) centre (0.0435, 77.6158) ccw